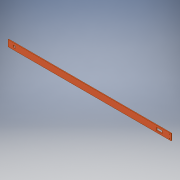
# Autodesk Inventor part: convyerwall
Saved by Autodesk Inventor 2019 (Build 230136000, 136)
## iProperties
Created: 2021-11-02
Part Number: convyerwall
Material: Generic
Document SubType Name: Modeling
Designer: modym
Density: 1 g/cm^3
Appearance: Smooth - Light Orange
Author: modym
Autodesk Inventor part; units mm, degrees
ref_plane "YZ Plane" through (0, 0, 0) normal (1, 0, 0) x (0, 1, 0)
ref_plane "XZ Plane" through (0, 0, 0) normal (0, 1, 0) x (-1, 0, 0)
ref_plane "XY Plane" through (0, 0, 0) normal (0, 0, 1) x (1, 0, 0)
sketch "Sketch1" plane through (0, 0, 0) normal (0, 0, 1) x (1, 0, 0)
  line L0 (0, 0) -> (1300, 0)
  line L1 (1300, 0) -> (1300, 50)
  line L2 (1300, 50) -> (0, 50)
  line L3 (0, 50) -> (0, 0)
  line L4 (0, 50) -> (50, 50)
  line L5 (50, 50) -> (50, 25)
  circle A0 centre (50, 25) radius 10.5
  line L6 (650, 50) -> (650, 17.5)
  circle A1 centre (1288, 40) radius 3
  circle A2 centre (1288, 10) radius 3
  line L7 (1182.5, 14.5) -> (1227.5, 14.5)
  line L8 (1227.5, 14.5) -> (1227.5, 35.5)
  line L9 (1227.5, 35.5) -> (1182.5, 35.5)
  line L10 (1182.5, 35.5) -> (1182.5, 14.5)
  dimension "d0" = 1300
  dimension "d1" = 50
  dimension "d4" = 50
  dimension "d5" = 21
  dimension "d10" = 6
  dimension "d11" = 6
  dimension "d14" = 45
  dimension "d17" = 21
  dimension "d18" = 14.5
  dimension "d19" = 25
  dimension "d20" = 12
  dimension "d21" = 12
  dimension "d22" = 10
  constraints: 22 end point, 4 parallel, 3 centre point, 3 perpendicular, 2 horizontal, 1 coincident, 1 midpoint, 1 point on line, 1 vertical
  measures "d0" distance of L2.end L1.end
  measures "d1" distance of L1.end L0.end
  measures "d4" distance of L2.end L4.end
  measures "d5" diameter of A0
  measures "d10" diameter of A1
  measures "d11" diameter of A2
  measures "d14" distance of L9.end L8.end
  measures "d17" distance of L7.end L8.end
  measures "d18" distance between parallel lines of L0 L7
  measures "d19" distance from line of L0 L5.end
  measures "d20" distance from line of L1 A1.centre
  measures "d21" distance from line of L1 A2.centre
  measures "d22" distance from line of L2 A1.centre
extrude "Extrusion4" add sketch "Sketch1" along normal blind 6
equation "\"d18\" = -0.5 * d17 + 0.5 * d1"
body "Solid4"
